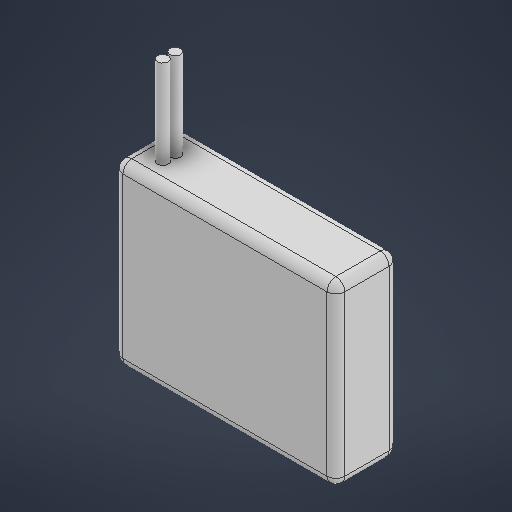
# Autodesk Inventor part: Bateria
Saved by Autodesk Inventor 2027 (Build 310192000, 192)
## iProperties
Created: 2026-06-25
Part Number: Bateria
Material: Genérico
Document SubType Name: Modeling
Designer: marcu
Density: 1 g/cm^3
Appearance: Padrão
Author: marcu
Autodesk Inventor part; units mm, degrees
ref_plane "YZ Plane" through (0, 0, 0) normal (1, 0, 0) x (0, 1, 0)
ref_plane "XZ Plane" through (0, 0, 0) normal (0, 1, 0) x (-1, 0, 0)
ref_plane "XY Plane" through (0, 0, 0) normal (0, 0, 1) x (1, 0, 0)
sketch "Esboço1" plane through (0, 0, 0) normal (0, 0, 1) x (1, 0, 0)
  line L0 (-12.5, 10) -> (12.5, 10)
  line L1 (12.5, 10) -> (12.5, -10)
  line L2 (12.5, -10) -> (-12.5, -10)
  line L3 (-12.5, -10) -> (-12.5, 10)
  line L4 (-12.5, 10) -> (12.5, -10) construction
  line L5 (12.5, 10) -> (-12.5, -10) construction
  point P0 (0, 0)
  dimension "d1" = 20
  dimension "d2" = 25
  constraints: 12 end point, 2 midpoint, 2 parallel, 1 horizontal, 1 perpendicular
  measures "d1" distance of L1.end L0.end
  measures "d2" distance of L0.end L0.start
extrude "Extrusão1" add sketch "Esboço1" along normal mid plane 7
fillet "Arredondamento1" radius 1 4 edges at (12.5, -10, 0) (-12.5, -10, 0) (12.5, 10, 0) (-12.5, 10, 0)
fillet "Arredondamento2" radius 1 16 edges at (12.2071, 9.7071, 3.5) (0, 10, 3.5) (-12.2071, 9.7071, 3.5) (-12.5, 0, 3.5) (-12.2071, -9.7071, 3.5) (0, -10, 3.5) (12.2071, -9.7071, 3.5) (12.5, 0, 3.5) (-12.2071, 9.7071, -3.5) (0, 10, -3.5) (12.2071, 9.7071, -3.5) (12.5, 0, -3.5) (12.2071, -9.7071, -3.5) (0, -10, -3.5) (-12.2071, -9.7071, -3.5) (-12.5, 0, -3.5)
sketch "Esboço6" plane through (-11.5, 10, -2.5) normal (0, 1, 0) x (1, 0, 0)
  circle A0 centre (2, -2.1) radius 0.6
  circle A1 centre (2, -3.5) radius 0.6
  line L0 (0, 0) -> (23, 0) projected
  line L1 (-1, -5) -> (0, -5) projected
  line L2 (0, 0) -> (0, -5) construction
  line L3 (23, -5) -> (0, -5) projected
  point P0 (11.5, -2.5)
  dimension "d24" = 1.2
  dimension "d25" = 2
  dimension "d26" = 2
  dimension "d27" = 1.5
  dimension "d28" = 1.5
  dimension "d29" = 0.2
  constraints: 2 centre point, 2 end point, 1 vertical
  measures "d24" diameter of A0
  measures "d25" distance from line of L2 A0.centre
  measures "d26" distance from line of L2 A1.centre
  measures "d27" distance from line of L3 A1.centre
  measures "d28" distance edge to line of A0 L0
extrude "Extrusão5" add sketch "Esboço6" along normal blind 10
